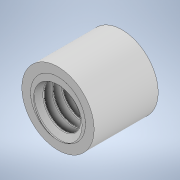
# Autodesk Inventor part: 8mmM6bushing
Saved by Autodesk Inventor 2020.2 (Build 242310000, 310)
## iProperties
Created: 2020-08-26
Part Number: 8mmM6bushing
Material: Generic
Document SubType Name: Modeling
Designer: elmar
Density: 1 g/cm^3
Appearance: Default
Author: elmar
Autodesk Inventor part; units mm, degrees
ref_plane "YZ Plane" through (0, 0, 0) normal (1, 0, 0) x (0, 1, 0)
ref_plane "XZ Plane" through (0, 0, 0) normal (0, 1, 0) x (-1, 0, 0)
ref_plane "XY Plane" through (0, 0, 0) normal (0, 0, 1) x (1, 0, 0)
sketch "Sketch1" plane through (0, 0, 0) normal (0, 0, 1) x (1, 0, 0)
  circle A0 centre (0, 0) radius 3.95
  dimension "d0" = 7.9
  constraints: 1 centre point, 1 coincident
  measures "d0" diameter of A0
extrude "Extrusion1" add sketch "Sketch1" along normal blind 7
sketch "Sketch2" plane through (0, 0, 0) normal (0, 0, -1) x (-1, 0, 0)
  point P0 (0, 0)
hole "Hole1" at (0, 0, 0) direction (0, 0, 1) diameter 6 end through all
thread "Thread1" size "M6x1" class "6H" standard "ANSI Metric M Profile" full length
sketch "Sketch4" plane through (0, 0, 0) normal (1, 0, 0) x (0, 1, 0)
  line L0 (3, 0) -> (3, 7)
  line L1 (3, 7) -> (2.2585, 7)
  line L2 (2.2585, 7) -> (2.2585, 0)
  line L3 (2.2585, 0) -> (3, 0)
  line L4 (0, -2.7086) -> (0, 8.6181) projected
  constraints: 8 end point
revolve "Revolution1" add sketch "Sketch4" angle 360 about axis through (0, 0, 0) along (0, 0, 1) separate body
sketch "Sketch3" plane through (0, 3, 0) normal (-1, 0, 0) x (0, 0, 1)
  line L0 (-0.5834, -0.0507) -> (-0.5001, -0.0507) construction
  line L1 (0.0832, -0.6911) -> (-0.0001, -0.8511) construction
  line L2 (-1.0001, -0.8511) -> (-1.0834, -0.6911) construction
  line L3 (-0.4168, -0.0507) -> (-0.5001, 0.1093) construction
  line L4 (-0.5001, 0.1093) -> (-0.5834, -0.0507) construction
  line L5 (-1.0001, -0.8511) -> (-0.9168, -0.6911) construction
  line L6 (-0.4168, -0.0507) -> (-0.0834, -0.6911)
  line L7 (-1.0834, -0.6911) -> (-0.9168, -0.6911) construction
  arc A0 (-1.0834, -0.6911) -> (-1.0001, -0.7416) centre (-1.0001, -0.6477) ccw construction
  line L8 (0.0832, -0.6911) -> (-0.0834, -0.6911) construction
  line L9 (-1.0001, -0.8511) -> (-1.0001, -0.6911) construction
  line L10 (-0.0001, -0.8511) -> (-0.0001, -0.6911) construction
  line L11 (-0.5001, 0.1093) -> (-0.5001, -0.0002) construction
  line L12 (-1.0001, -0.7416) -> (-0.0001, -0.7416)
  arc A1 (-1.0001, -0.7416) -> (-0.9168, -0.6911) centre (-1.0001, -0.6477) ccw
  line L13 (-0.0834, -0.6911) -> (-0.0001, -0.8511) construction
  line L14 (-0.9168, -0.6911) -> (-0.5834, -0.0507)
  line L15 (-0.0001, -0.0002) -> (-0.0001, 0.0177)
  line L16 (-0.0001, 0.0177) -> (-0.0001, -0.0002)
  line L17 (-0.0001, -0.0002) -> (0.0334, -0.0002)
  arc A2 (-0.0834, -0.6911) -> (-0.0001, -0.7416) centre (-0.0001, -0.6477) ccw
  arc A3 (-0.0001, -0.7416) -> (0.0832, -0.6911) centre (-0.0001, -0.6477) ccw construction
  arc A4 (-0.5001, -0.0002) -> (-0.5834, -0.0507) centre (-0.5001, -0.0941) ccw
  arc A5 (-0.4168, -0.0507) -> (-0.5001, -0.0002) centre (-0.5001, -0.0941) ccw
  line L18 (-0.5001, -0.0002) -> (-0.5001, -0.0507) construction
  line L19 (-0.5001, -0.0507) -> (-0.4168, -0.0507) construction
  dimension "d12" = 55
  dimension "d13" = 0.1601
  dimension "d14" = 0.1601
  dimension "Sketch3_ThreadOffset" = 0
  dimension "Sketch3_MajorRadius" = 0.7415
  dimension "d17" = 1
  dimension "Sketch3_MinorRadius" = 0
  constraints: 40 end point, 12 point on circle, 10 parallel, 8 tangent, 6 centre point, 6 collinear, 2 midpoint, 2 point on line, 1 horizontal, 1 perpendicular, 3 other
  measures "d12" angle of L6 L14
  measures "d13" distance of L3.end L0.end
  measures "d14" distance of L1.end L10.end
  measures "Sketch3_ThreadOffset" distance between parallel lines of L15 L10
  measures "Sketch3_MajorRadius" distance from line of L12 L15.start
  measures "d17" distance from line of L1.end L9
  measures "Sketch3_MinorRadius" distance edge to line of A5 L17
coil "Coil1" sketch "Sketch3" operation cut axis through (0, 0, 0) along (0, 0, 1) pitch 1.001 turns 8.991009 hand right bodies 2
equation "\"d12\" = d19"
equation "\"d13\" = 0.160083 * Sketch3_Pitch"
equation "\"d14\" = 0.160083 * Sketch3_Pitch"
equation "\"d17\" = Sketch3_Pitch"
equation "\"d19\" = 55deg"
equation "\"Sketch3_Pitch\" = 1"
body "Solid1"
body "Solid2"
